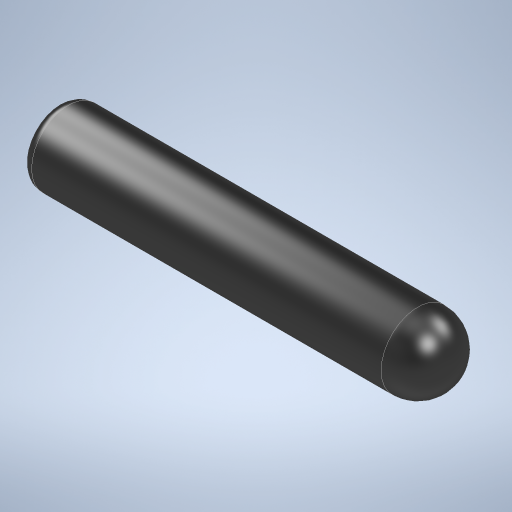
# Autodesk Inventor part: Stift_lang
Saved by Autodesk Inventor 2024 (Build 280153000, 153)
## iProperties
Created: 2023-08-24
Part Number: Stift_lang
Material: Generisch
Document SubType Name: Modeling
Designer: rapp
Density: 1 g/cm^3
Appearance: Glänzend - Schwarz
Author: rapp
Autodesk Inventor part; units mm, degrees
ref_plane "YZ Plane" through (0, 0, 0) normal (1, 0, 0) x (0, 1, 0)
ref_plane "XZ Plane" through (0, 0, 0) normal (0, 1, 0) x (-1, 0, 0)
ref_plane "XY Plane" through (0, 0, 0) normal (0, 0, 1) x (1, 0, 0)
sketch "Skizze1" plane through (0, 0, 0) normal (0, 0, 1) x (1, 0, 0)
  line L0 (-11.0071, 0) -> (66.0426, 0) projected
  line L1 (0, -1.2071) -> (0, 7.2426) projected
  line L2 (0, 0) -> (54, 0)
  line L3 (49, 5) -> (0, 5)
  line L4 (0, 5) -> (0, 0)
  arc A0 (54, 0) -> (49, 5) centre (49, 0) ccw
  point P0 (54, 0)
  dimension "d0" = 49
  dimension "d1" = 10
  constraints: 6 end point, 2 point on circle, 1 centre point, 1 horizontal, 1 parallel
  measures "d0" distance of L3.end L3.start
  measures "d1" diameter of L3 L0
revolve "Umdrehung1" add sketch "Skizze1" angle 360 about axis through (-10, 0, 0) along (1, 0, 0)
fillet "Rundung1" radius 1.5 1 edges at (0, -5, 0)
